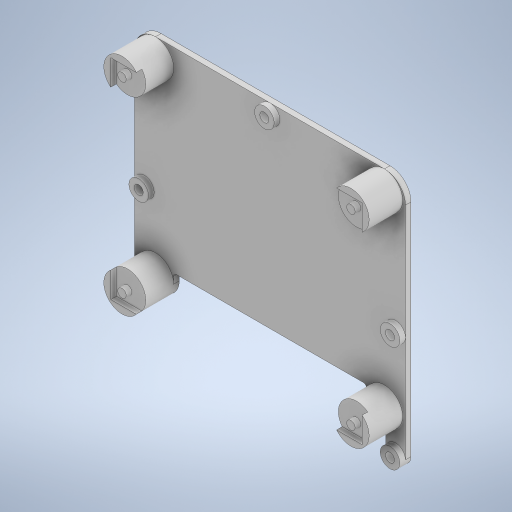
# Autodesk Inventor part: 3D_Druck_Teil_V2
Saved by Autodesk Inventor 2023 (Build 270158000, 158)
## iProperties
Created: 2022-12-01
Part Number: 3D_Druck_Teil_V2
Material: Generisch
Document SubType Name: Modeling
Designer: Admin
Density: 1 g/cm^3
Appearance: Vorgabe
Author: Admin
Autodesk Inventor part; units mm, degrees
ref_plane "YZ Plane" through (0, 0, 0) normal (1, 0, 0) x (0, 1, 0)
ref_plane "XZ Plane" through (0, 0, 0) normal (0, 1, 0) x (-1, 0, 0)
ref_plane "XY Plane" through (0, 0, 0) normal (0, 0, 1) x (1, 0, 0)
sketch "Skizze1" plane through (0, 0, 0) normal (0, 0, 1) x (1, 0, 0)
  line L0 (0, 0) -> (97, 0)
  line L1 (97, 0) -> (97, 80)
  line L2 (97, 80) -> (0, 80)
  line L3 (0, 80) -> (0, 0)
  dimension "d1" = 80
  dimension "d2" = 97
  constraints: 8 end point, 2 parallel, 1 horizontal, 1 perpendicular
  measures "d1" distance between parallel lines of L0 L2
  measures "d2" distance of L1.end L2.end
extrude "Extrusion1" add sketch "Skizze1" along normal blind 2
sketch "Skizze2" plane through (0, 0, 2) normal (0, 0, 1) x (1, 0, 0)
  line L0 (7.5, 73.5) -> (89.5, 73.5) construction
  line L1 (89.5, 73.5) -> (89.5, 6.5) construction
  line L2 (89.5, 6.5) -> (7.5, 6.5) construction
  line L3 (7.5, 6.5) -> (7.5, 73.5) construction
  line L4 (48.5, 73.5) -> (48.5, 80) construction
  line L5 (97, 80) -> (0, 80) projected
  line L6 (89.5, 40) -> (97, 40) construction
  line L7 (97, 0) -> (97, 80) projected
  line L8 (48.5, 6.5) -> (48.5, 0) construction
  line L9 (0, 0) -> (97, 0) projected
  line L10 (7.5, 40) -> (0, 40) construction
  line L11 (0, 80) -> (0, 0) projected
  circle A0 centre (7.5, 73.5) radius 6.5
  circle A1 centre (89.5, 73.5) radius 6.5
  circle A2 centre (89.5, 6.5) radius 6.5
  circle A3 centre (7.5, 6.5) radius 6.5
  dimension "d5" = 82
  dimension "d6" = 67
  dimension "d7" = 13
  constraints: 16 end point, 8 midpoint, 4 centre point, 4 coincident, 3 equal radius, 2 horizontal, 2 parallel, 1 perpendicular, 1 vertical
  measures "d5" distance of L0.start L0.end
  measures "d6" distance of L0.end L1.end
  measures "d7" diameter of A0
extrude "Extrusion2" add sketch "Skizze2" along normal blind 12 contours A1 | A0 | A3 | A2
sketch "Skizze3" plane through (89.5, 73.5, 14) normal (0, 0, 1) x (1, 0, 0)
  line L0 (-86, 4) -> (4, 4)
  line L1 (4, 4) -> (4, -71)
  line L2 (4, -71) -> (-86, -71)
  line L3 (-86, -71) -> (-86, 4)
  line L4 (-41, -71) -> (-41, -73.5)
  line L5 (-89.5, -73.5) -> (7.5, -73.5) projected
  line L6 (4, -33.5) -> (7.5, -33.5)
  line L7 (7.5, -73.5) -> (7.5, 6.5) projected
  line L8 (-89.5, 6.5) -> (-89.5, -73.5) projected
  line L9 (-89.5, -33.5) -> (-86, -33.5)
  line L10 (-41, 4) -> (-41, 6.5)
  line L11 (7.5, 6.5) -> (-89.5, 6.5) projected
  circle A0 centre (-82, 0) radius 6.5 projected
  circle A1 centre (0, -67) radius 6.5 projected
  circle A2 centre (-82, -67) radius 6.5 projected
  point P0 (-85, -5.7663)
  point P1 (-85, 5.7663)
  point P2 (-88.5, 0)
  point P3 (-82, 6.5)
  dimension "d10" = 75
  dimension "d11" = 90
  constraints: 16 end point, 7 midpoint, 2 horizontal, 2 parallel, 1 perpendicular, 1 point on line, 1 vertical, 2 other
  measures "d10" distance of L2.end L0.start
  measures "d11" distance of L0.start L0.end
extrude "Extrusion3" cut sketch "Skizze3" against normal blind 2 contours L0 L1 A1 L2 A2 L3 A0 | A0 L3 L0 | L1 L2 A1 | A2 L2 L3 picked at (-80.5561, -1.9495) picked at (-1.3202, -64.9474) picked at (-80.5561, -65.0505)
sketch "Skizze4" plane through (89.5, 73.5, 12) normal (0, 0, 1) x (1, 0, 0)
  circle A0 centre (-82, 0) radius 6.5 projected
  circle A1 centre (-82, 0) radius 1.5
  circle A2 centre (0, 0) radius 6.5 projected
  circle A3 centre (0, 0) radius 1.5
  circle A4 centre (-82, -67) radius 6.5 projected
  circle A5 centre (-82, -67) radius 1.5
  arc A6 (4, -61.8765) -> (-5.1235, -71) centre (0, -67) ccw projected
  circle A7 centre (0, -67) radius 1.5
  point P0 (-89.5, -73.5)
  point P1 (-85, -5.7663)
  point P2 (-85, 5.7663)
  point P3 (3, 5.7663)
  point P4 (3, -5.7663)
  point P5 (-85, -72.7663)
  point P6 (-85, -61.2337)
  point P7 (-88.5, 0)
  point P8 (-82, 6.5)
  point P9 (6.5, 0)
  point P10 (0, 6.5)
  point P11 (-82, -73.5)
  point P12 (-88.5, -67)
  dimension "d15" = 3
  constraints: 4 centre point, 4 coincident, 3 equal radius
  measures "d15" diameter of A1
extrude "Extrusion4" add sketch "Skizze4" along normal up to surface (2 mm away) contours A1 | A3 | A5 | A7
sketch "Skizze9" plane through (0, 0, 2) normal (0, 0, 1) x (1, 0, 0)
  line L0 (0, 0) -> (97, 0) projected
  line L1 (14, 0) -> (83, 0)
  line L2 (83, 0) -> (83, 10)
  line L3 (83, 10) -> (14, 10)
  line L4 (14, 10) -> (14, 0)
  line L5 (48.5, 10) -> (48.5, 0)
  point P0 (83, 0)
  dimension "d39" = 10
  dimension "d40" = 69
  constraints: 10 end point, 2 midpoint, 2 parallel, 1 horizontal, 1 perpendicular, 1 point on line, 1 vertical
  measures "d39" distance of L3.end L1.start
  measures "d40" distance of L2.end L3.end
extrude "Extrusion7" cut sketch "Skizze9" against normal blind 2
sketch "Skizze7" plane through (0, 0, 2) normal (0, 0, 1) x (1, 0, 0)
  line L0 (97, 0) -> (97, 80) projected
  line L1 (90, 0) -> (90, -6.5)
  line L2 (97, -6.5) -> (97, 0)
  arc A0 (90, -6.5) -> (97, -6.5) centre (93.5, -6.5) ccw
  line L3 (90, 0) -> (97, 0)
  line L4 (0, 0) -> (97, 0) projected
  point P0 (89.5, 0)
  dimension "d31" = 7
  dimension "d47" = 0
  dimension "d48" = 6.5
  constraints: 6 end point, 2 point on circle, 2 tangent, 1 centre point, 1 collinear, 1 horizontal, 1 parallel, 1 vertical
  measures "d31" distance between parallel lines of L2 L1
  measures "d47" distance between parallel lines of L0 L2
  measures "d48" distance from line of L3 A0.centre
extrude "Extrusion6" add sketch "Skizze7" against normal up to surface (2 mm away)
sketch "Skizze5" plane through (0, 0, 2) normal (0, 0, 1) x (1, 0, 0)
  line L0 (48.5, 76.5) -> (48.5, 0)
  line L1 (93.5, 31.5) -> (93.5, -6.5)
  line L2 (0, 0) -> (97, 0) projected
  point P0 (3.5, 31.5)
  point P1 (7.5, 0)
  point P2 (89.5, 0)
  dimension "d18" = 90
  dimension "d19" = 38
  dimension "d30" = 31.5
  dimension "d37" = 45
  constraints: 4 end point, 2 vertical, 1 coincident, 1 midpoint, 1 symmetric about line
  measures "d18" distance of L1.start point (3.5, 31.5)
  measures "d19" distance of L1.start L1.end
  measures "d30" distance from line of L2 point (3.5, 31.5)
  measures "d37" horizontal distance of point (48.5, 76.5) point (3.5, 31.5)
hole "Bohrung1" at (3.5, 31.5, 2) at (93.5, 31.5, 2) at (93.5, -6.5, 2) at (48.5, 76.5, 2) direction (0, 0, -1) diameter 3.2 end through all
sketch "Skizze6" plane through (0, 0, 2) normal (0, 0, 1) x (1, 0, 0)
  circle A0 centre (3.5, 31.5) radius 1.6 projected
  circle A1 centre (93.5, 31.5) radius 1.6 projected
  circle A2 centre (93.5, -6.5) radius 1.6 projected
  circle A3 centre (93.5, -6.5) radius 1.6
  circle A4 centre (93.5, 31.5) radius 1.6
  circle A5 centre (3.5, 31.5) radius 1.6
  circle A6 centre (48.5, 76.5) radius 1.6 projected
  circle A7 centre (48.5, 76.5) radius 1.5
  circle A8 centre (48.5, 76.5) radius 3.5
  circle A9 centre (3.5, 31.5) radius 3.5
  circle A10 centre (93.5, 31.5) radius 3.5
  circle A11 centre (93.5, -6.5) radius 3.5
  point P0 (0, 0)
  point P1 (0, 42.882)
  point P2 (0, 45.118)
  point P3 (88, 45.118)
  point P4 (88, 42.882)
  point P5 (88, 0.118)
  point P6 (87.882, 0)
  dimension "d45" = 7
  constraints: 8 centre point, 7 coincident, 3 equal radius, 6 other
  measures "d45" diameter of A8
extrude "Extrusion5" add sketch "Skizze6" along normal blind 2 and the other way blind 2 contours A8 | A9 | A10 | A11
fillet "Rundung1" radius 7.5 3 edges at (97, 80, 1) (0, 80, 1) (0, 0, 1)
fillet "Rundung2" radius 1 3 edges at (90, 0, 1) (83, 10, 1) (14, 10, 1)
fillet "Rundung3" radius 6.5 2 edges at (83, 0, 1) (14, 0, 1)
sketch "Skizze10" plane through (0, 0, 0) normal (0, 0, -1) x (-1, 0, 0)
  point P0 (0, 0)
